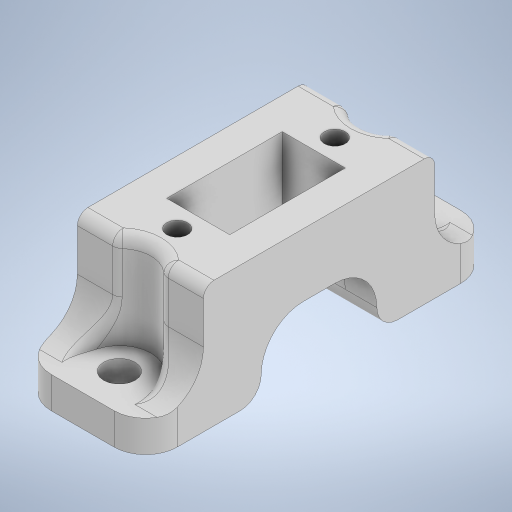
# Autodesk Inventor part: switchPilot
Saved by Autodesk Inventor 2023 (Build 270158000, 158)
## iProperties
Created: 2023-12-12
Part Number: switchPilot
Material: Generic
Document SubType Name: Modeling
Designer: Dawid
Density: 1 g/cm^3
Appearance: Default
Author: Dawid
Autodesk Inventor part; units mm, degrees
ref_plane "YZ Plane" through (0, 0, 0) normal (1, 0, 0) x (0, 1, 0)
ref_plane "XZ Plane" through (0, 0, 0) normal (0, 1, 0) x (-1, 0, 0)
ref_plane "XY Plane" through (0, 0, 0) normal (0, 0, 1) x (1, 0, 0)
sketch "Sketch1" plane through (0, 0, 0) normal (0, 1, 0) x (-1, 0, 0)
  line L0 (3, 5.5) -> (-3, 5.5)
  line L1 (-3, 5.5) -> (-3, -5.5)
  line L2 (-3, -5.5) -> (3, -5.5)
  line L3 (3, -5.5) -> (3, 5.5)
  line L4 (3, 5.5) -> (-3, -5.5) construction
  line L5 (-3, 5.5) -> (3, -5.5) construction
  line L6 (-6, 11) -> (6, 11)
  line L7 (6, 11) -> (6, -11)
  line L8 (6, -11) -> (-6, -11)
  line L9 (-6, -11) -> (-6, 11)
  line L10 (-6, 11) -> (6, -11) construction
  line L11 (6, 11) -> (-6, -11) construction
  line L12 (0, 0) -> (0, 7.5)
  line L13 (0, 7.5) -> (0, -7.5)
  circle A0 centre (0, 7.5) radius 1
  circle A1 centre (0, -7.5) radius 1
  dimension "d0" = 6
  dimension "d1" = 11
  dimension "d2" = 12
  dimension "d3" = 22
  dimension "d4" = 7.5
  dimension "d5" = 15
  dimension "d6" = 2
  dimension "d7" = 2
  constraints: 28 end point, 4 midpoint, 4 parallel, 2 centre point, 2 coincident, 2 horizontal, 2 perpendicular, 1 point on line, 1 vertical
  measures "d0" distance of L2.end L1.end
  measures "d1" distance of L1.end L0.end
  measures "d2" distance of L7.end L8.end
  measures "d3" distance of L6.end L7.end
  measures "d4" distance of L12.start L12.end
  measures "d5" distance of L12.end L13.end
  measures "d6" diameter of A0
  measures "d7" diameter of A1
extrude "Extrusion1" add sketch "Sketch1" along normal blind 6
sketch "Sketch2" plane through (0, 0, 0) normal (0, -1, 0) x (1, 0, 0)
  line L0 (6, -11) -> (-6, -11) projected
  line L1 (6, 11) -> (-6, 11)
  line L2 (-6, 11) -> (-6, -11)
  line L3 (-6, -11) -> (6, -11)
  line L4 (6, -11) -> (6, 11)
  line L5 (6, 11) -> (-6, -11) construction
  line L6 (-6, 11) -> (6, -11) construction
  line L7 (-3, 5.5) -> (-3, -5.5) projected
  line L8 (3, 5.5) -> (-3, 5.5)
  line L9 (-3, 5.5) -> (-3, -5.5)
  line L10 (-3, -5.5) -> (3, -5.5)
  line L11 (3, -5.5) -> (3, 5.5)
  line L12 (3, 5.5) -> (-3, -5.5) construction
  line L13 (-3, 5.5) -> (3, -5.5) construction
  line L14 (3, 5.5) -> (6, 5.5)
  line L15 (6, 11) -> (6, -11) projected
  line L16 (-3, -5.5) -> (3, -5.5) projected
  line L17 (3, -5.5) -> (6, -5.5)
  line L18 (-3, -5.5) -> (-6, -5.5)
  line L19 (-6, -11) -> (-6, 11) projected
  line L20 (3, 5.5) -> (-3, 5.5) projected
  line L21 (-3, 5.5) -> (-6, 5.5)
  point P0 (0, 0)
  constraints: 32 end point, 6 point on line, 4 midpoint, 4 parallel, 4 perpendicular, 2 horizontal
extrude "Extrusion2" add sketch "Sketch2" along normal blind 6 contours L0 L2 L18 L10 L17 L4 | L14 L8 L21 L2 L1 L4
sketch "Sketch3" plane through (6, 0, 5.5) normal (1, 0, 0) x (0, 0, -1)
  line L0 (11, -6) -> (16.5, -6) projected
  line L1 (11, -6) -> (22, -6)
  line L2 (22, -6) -> (22, -3)
  line L3 (22, -3) -> (11, -3)
  line L4 (11, -3) -> (11, -6)
  line L5 (0, -6) -> (-5.5, -6) projected
  line L6 (0, -6) -> (-11, -6)
  line L7 (-11, -6) -> (-11, -3)
  line L8 (-11, -3) -> (0, -3)
  line L9 (0, -3) -> (0, -6)
  point P0 (5.5, 0)
  dimension "d12" = 11
  dimension "d13" = 3
  dimension "d14" = 11
  dimension "d15" = 3
  constraints: 16 end point, 4 parallel, 2 horizontal, 2 perpendicular
  measures "d12" distance of L3.end L2.end
  measures "d13" distance of L2.end L1.end
  measures "d14" distance of L7.end L8.end
  measures "d15" distance of L6.end L7.end
extrude "Extrusion3" add sketch "Sketch3" against normal blind 12
sketch "Sketch4" plane through (0, -6, 0) normal (0, -1, 0) x (1, 0, 0)
  line L0 (6, -16.5) -> (-6, -16.5) projected
  line L1 (-6, -16.5) -> (0, -16.5)
  line L2 (0, -16.5) -> (0, -13)
  line L3 (-6, 5.5) -> (-6, 16.5) projected
  line L4 (-6, 16.5) -> (0, 16.5)
  line L5 (6, 16.5) -> (-6, 16.5) projected
  line L6 (0, 16.5) -> (0, 13)
  circle A0 centre (0, -13) radius 1.5
  circle A1 centre (0, 13) radius 1.5
  point P0 (0, 0)
  dimension "d18" = 3.5
  dimension "d19" = 3.5
  dimension "d20" = 3
  dimension "d21" = 3
  constraints: 8 end point, 2 centre point, 2 coincident, 2 midpoint, 2 perpendicular
  measures "d18" distance of L1.end L2.end
  measures "d19" distance of L4.end L6.end
  measures "d20" diameter of A0
  measures "d21" diameter of A1
extrude "Extrusion4" cut sketch "Sketch4" against normal blind 12
sketch "Sketch5" plane through (6, -3, -11) normal (0, 1, 0) x (1, 0, 0)
  circle A0 centre (-6, 2) radius 1.5 projected
  circle A1 centre (-6, 2) radius 3
  circle A2 centre (-6, -24) radius 1.5 projected
  circle A3 centre (-6, -24) radius 3
  point P0 (-6, -11)
  dimension "d24" = 6
  dimension "d25" = 6
  constraints: 2 centre point, 2 coincident
  measures "d24" diameter of A1
  measures "d25" diameter of A3
extrude "Extrusion5" cut sketch "Sketch5" along normal blind 12
fillet "Fillet1" radius 4 4 edges at (-4.5, 0, 5.5) (4.5, 0, 5.5) (4.5, 0, -5.5) (-4.5, 0, -5.5)
fillet "Fillet2" radius 3 4 edges at (6, -4.5, -16.5) (6, -4.5, 16.5) (-6, -4.5, 16.5) (-6, -4.5, -16.5)
fillet "Fillet3" radius 4 4 edges at (4.118, -3, 11) (-4.118, -3, 11) (-4.118, -3, -11) (4.118, -3, -11)
fillet "Fillet4" radius 1 8 edges at (-2.8457, -1.7015, -12.0501) (-2.2361, 3.5, -11) (2.8448, -1.6988, -12.0477) (2.2361, 3.5, -11) (-2.2361, 3.5, 11) (-2.8457, -1.7016, 12.0502) (2.2361, 3.5, 11) (2.9543, -2.1053, 12.4786)
fillet "Fillet5" radius 1 10 edges at (-2.2922, 6, -10.9354) (0, 6, -10) (2.2922, 6, -10.9354) (4.3229, 6, -11) (-4.3229, 6, -11) (-2.2922, 6, 10.9354) (0, 6, 10) (2.2922, 6, 10.9354) (4.3229, 6, 11) (-4.3229, 6, 11)
fillet "Fillet6" radius 2 2 edges at (0, -6, -5.5) (0, -6, 5.5)
body "Solid1"
